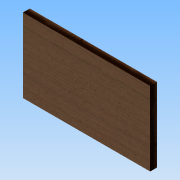
# Autodesk Inventor part: cache
Saved by Autodesk Inventor 2015 (Build 190159000, 159)
## iProperties
Created: 2015-12-28
Part Number: cache
Material: Générique
Document SubType Name: Modeling
Designer: Gregwar
Density: 1 g/cm^3
Appearance: Par défaut
Author: Gregwar
Autodesk Inventor part; units mm, degrees
ref_plane "YZ Plane" through (0, 0, 0) normal (1, 0, 0) x (0, 1, 0)
ref_plane "XZ Plane" through (0, 0, 0) normal (0, 1, 0) x (-1, 0, 0)
ref_plane "XY Plane" through (0, 0, 0) normal (0, 0, 1) x (1, 0, 0)
sketch "Esquisse1" plane through (0, 0, 0) normal (0, 1, 0) x (-1, 0, 0)
  line L0 (0, 0) -> (55, 0)
  line L1 (55, 0) -> (55, -32)
  line L2 (55, -32) -> (0, -32)
  line L3 (0, -32) -> (0, 0)
  line L4 (55, -16) -> (0, -16) construction
  line L5 (0, -32) -> (5, -32)
  line L6 (55, 0) -> (0, 0)
  line L7 (0, 0) -> (0, -32)
  line L8 (0, 0) -> (5, 0)
  dimension "d0" = 32
  dimension "d6" = 55
  constraints: 18 end point, 2 horizontal, 2 midpoint, 2 parallel, 2 symmetric about line, 1 perpendicular
  measures "d0" distance of L2.end L0.start
  measures "d6" distance of L1.end L2.end
extrude "Extrusion1" add sketch "Esquisse1" along normal blind 3
